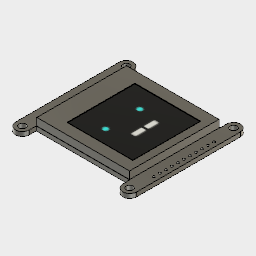
2088 1.44in TFT Display (Autodesk Fusion 360 design; units mm, degrees)
Autodesk Fusion 360 part; units mm, degrees
sketch "Adafruit TFT144 Breakout rev B" plane through (0, 0, 0) normal (0, 0, 1) x (1, 0, 0)
  line L0 (5.08, 33.02) -> (5.08, 35.56)
  arc A0 (2.54, 38.1) -> (0, 35.56) centre (2.54, 35.56) ccw
  line L1 (5.08, 0) -> (39.37, 0)
  arc A1 (0, -2.54) -> (2.54, -5.08) centre (2.54, -2.54) ccw
  arc A2 (44.45, 35.56) -> (41.91, 38.1) centre (41.91, 35.56) ccw
  line L2 (39.37, 33.02) -> (5.08, 33.02)
  arc A3 (39.37, -2.54) -> (41.91, -5.08) centre (41.91, -2.54) ccw
  arc A4 (5.08, 35.56) -> (2.54, 38.1) centre (2.54, 35.56) ccw
  line L3 (5.08, -2.54) -> (5.08, 0)
  arc A5 (41.91, 38.1) -> (39.37, 35.56) centre (41.91, 35.56) ccw
  arc A6 (41.91, -5.08) -> (44.45, -2.54) centre (41.91, -2.54) ccw
  line L4 (39.37, 35.56) -> (39.37, 33.02)
  line L5 (44.45, -2.54) -> (44.45, 35.56)
  line L6 (0, 35.56) -> (0, -2.54)
  line L7 (39.37, 0) -> (39.37, -2.54)
  arc A7 (2.54, -5.08) -> (5.08, -2.54) centre (2.54, -2.54) ccw
  circle A8 centre (2.54, 35.56) radius 1.25
  circle A9 centre (41.91, 35.56) radius 1.25
  circle A10 centre (2.54, -2.54) radius 1.25
  circle A11 centre (41.91, -2.54) radius 1.25
  line L8 (44.45, 16.51) -> (0, 16.51) construction
  circle A12 centre (42.75, 27.51) radius 0.45
  circle A13 centre (42.75, 25.31) radius 0.45
  circle A14 centre (42.75, 23.11) radius 0.45
  circle A15 centre (42.75, 20.91) radius 0.45
  circle A16 centre (42.75, 18.71) radius 0.45
  circle A17 centre (42.75, 16.51) radius 0.45
  circle A18 centre (42.75, 14.31) radius 0.45
  circle A19 centre (42.75, 12.11) radius 0.45
  circle A20 centre (42.75, 9.91) radius 0.45
  circle A21 centre (42.75, 7.71) radius 0.45
  circle A22 centre (42.75, 5.51) radius 0.45
  dimension "d3" = 2.5
  dimension "d4" = 2.5
  dimension "d5" = 2.5
  dimension "d6" = 2.5
  dimension "d25" = 0.9
  dimension "d26" = 1.7
  dimension "d29" = 0
  dimension "d30" = -2.2
  measures "d3" diameter of A8
  measures "d4" diameter of A9
  measures "d5" diameter of A10
  measures "d6" diameter of A11
  measures "d25" diameter of A12
  measures "d26" distance of L5 A12.centre
extrude "Extrude1" add sketch "Adafruit TFT144 Breakout rev B" along normal blind 1.6 contours L0 A0 L1 A1 A2 L2 A3 A4 L3 A5 A6 L4 L5 L6 L7 A7 | A12 | A13 | A14 | A15 | A16 | A17 | A18 | A19 | A20 | A21 | A22 makes body 1
sketch "Display Glass" plane through (0, 0, 1.6) normal (0, 0, 1) x (-1, 0, 0)
  circle A0 centre (-41.91, -35.56) radius 1.25
  circle A1 centre (-41.91, 2.54) radius 1.25
  circle A2 centre (-2.54, 2.54) radius 1.25
  circle A3 centre (-2.54, -35.56) radius 1.25
  arc A4 (0, 2.54) -> (-5.08, 2.54) centre (-2.54, 2.54) ccw
  line L0 (-5.08, 2.54) -> (-5.08, 0)
  line L1 (-5.08, 0) -> (-39.37, 0)
  line L2 (-39.37, 0) -> (-39.37, 2.54)
  arc A5 (-39.37, 2.54) -> (-44.45, 2.54) centre (-41.91, 2.54) ccw
  line L3 (-44.45, 2.54) -> (-44.45, -35.56)
  arc A6 (-44.45, -35.56) -> (-39.37, -35.56) centre (-41.91, -35.56) ccw
  line L4 (-39.37, -35.56) -> (-39.37, -33.02)
  line L5 (-39.37, -33.02) -> (-5.08, -33.02)
  line L6 (-5.08, -33.02) -> (-5.08, -35.56)
  arc A7 (-5.08, -35.56) -> (0, -35.56) centre (-2.54, -35.56) ccw
  line L7 (0, -35.56) -> (0, 2.54)
  line L8 (-5.225, -32.94) -> (-39.225, -32.94)
  line L9 (-39.225, -32.94) -> (-39.225, -0.08)
  line L10 (-39.225, -0.08) -> (-5.225, -0.08)
  line L11 (-5.225, -0.08) -> (-5.225, -32.94)
  line L12 (-5.225, -16.51) -> (-39.225, -16.51) construction
  line L13 (-22.225, -32.94) -> (-22.225, -0.08) construction
  line L14 (0, -16.51) -> (-44.45, -16.51) construction
  line L15 (-22.225, -33.02) -> (-22.225, 0) construction
  dimension "d9" = 34
  dimension "d10" = 32.86
  measures "d9" distance of L8.start L8.end
  measures "d10" distance of L8.start L10.end
extrude "Extrude2" add sketch "Display Glass" along normal blind 2.74 separate body contours L8 L9 L10 L11 makes body 2
sketch "Display View" plane through (0, 0, 4.34) normal (0, 0, 1) x (-1, 0, 0)
  line L0 (-5.225, -0.08) -> (-39.225, -0.08)
  line L1 (-39.225, -0.08) -> (-39.225, -32.94)
  line L2 (-39.225, -32.94) -> (-5.225, -32.94)
  line L3 (-5.225, -32.94) -> (-5.225, -0.08)
  line L4 (-12.325, -28.94) -> (-36.425, -28.94)
  line L5 (-36.425, -28.94) -> (-36.425, -4.08)
  line L6 (-36.425, -4.08) -> (-12.325, -4.08)
  line L7 (-12.325, -4.08) -> (-12.325, -28.94)
  dimension "d13" = 2.8
  dimension "d14" = 7.1
  dimension "d15" = 4
  dimension "d16" = 4
  measures "d13" distance of L1 L5
  measures "d14" distance of L3 L7
  measures "d15" distance of L2 L4
  measures "d16" distance of L0 L6
extrude "Extrude3" cut sketch "Display View" against normal blind 0.2 contours L4 L5 L6 L7 bodies 2
sketch "microSD" plane through (0, 0, 0) normal (0, 0, -1) x (1, 0, 0)
  circle A0 centre (41.91, -35.56) radius 1.25
  circle A1 centre (41.91, 2.54) radius 1.25
  circle A2 centre (2.54, 2.54) radius 1.25
  circle A3 centre (2.54, -35.56) radius 1.25
  arc A4 (5.08, 2.54) -> (0, 2.54) centre (2.54, 2.54) ccw
  line L0 (0, 2.54) -> (0, -35.56)
  arc A5 (0, -35.56) -> (5.08, -35.56) centre (2.54, -35.56) ccw
  line L1 (5.08, -35.56) -> (5.08, -33.02)
  line L2 (5.08, -33.02) -> (39.37, -33.02)
  line L3 (39.37, -33.02) -> (39.37, -35.56)
  arc A6 (39.37, -35.56) -> (44.45, -35.56) centre (41.91, -35.56) ccw
  line L4 (44.45, -35.56) -> (44.45, 2.54)
  arc A7 (44.45, 2.54) -> (39.37, 2.54) centre (41.91, 2.54) ccw
  line L5 (39.37, 2.54) -> (39.37, 0)
  line L6 (39.37, 0) -> (5.08, 0)
  line L7 (5.08, 0) -> (5.08, 2.54)
  line L8 (0.829, -22.733) -> (16.129, -22.733)
  line L9 (16.129, -22.733) -> (16.129, -8.733)
  line L10 (16.129, -8.733) -> (0.829, -8.733)
  line L11 (0.829, -8.733) -> (0.829, -22.733)
  spline S0 degree 2 poles (0.829, -8.733) (3.3168, -15.733) (0.829, -22.733) knots 0 0 0 1.414905 1.414905 1.414905 weights 1 0.699738 1
  dimension "d19" = 15.3
  dimension "d20" = 14
  dimension "d21" = 22.733
  dimension "d22" = 16.129
  measures "d19" distance of L8.start L8.end
  measures "d20" distance of L8.start L10.end
  measures "d21" distance of origin L8
  measures "d22" distance of origin L9
extrude "Extrude4" add sketch "microSD" along normal blind 1.8 separate body contours L8 L9 L10 S0 makes body 3
extrude "Extrude5" cut sketch "Adafruit TFT144 Breakout rev B" along normal up to surface (1.6 mm away) contours A12 | A13 | A14 | A15 | A16 | A17 | A18 | A19 | A20 | A21 | A22 bodies 1
named bodies: "PCB", "Display", "microSD"
